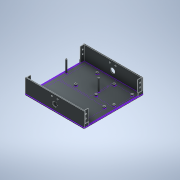
# Autodesk Inventor part: Lower_Housing
Saved by Autodesk Inventor 2022 (Build 260153000, 153)
## iProperties
Created: 2022-03-06
Part Number: Lower_Housing
Material: Iron, Cast
Document SubType Name: Modeling
Designer: Hajar
Density: 7.15 g/cm^3
Appearance: Iron Gray
Author: Hajar
Autodesk Inventor part; units mm, degrees
ref_plane "YZ Plane" through (0, 0, 0) normal (1, 0, 0) x (0, 1, 0)
ref_plane "XZ Plane" through (0, 0, 0) normal (0, 1, 0) x (-1, 0, 0)
ref_plane "XY Plane" through (0, 0, 0) normal (0, 0, 1) x (1, 0, 0)
sketch "Sketch1" plane through (0, 0, 0) normal (0, 1, 0) x (-1, 0, 0)
  line L0 (101.0364, -60.995) -> (-18.9636, -60.995)
  line L1 (-18.9636, -60.995) -> (-18.9636, 59.005)
  line L2 (-18.9636, 59.005) -> (101.0364, 59.005)
  line L3 (101.0364, 59.005) -> (101.0364, -60.995)
  line L4 (93.1598, 54.938) -> (-8.3402, 54.938) construction
  line L5 (-8.3402, 54.938) -> (-8.3402, 1.138) construction
  line L6 (-8.3402, 1.138) -> (93.1598, 1.138) construction
  line L7 (93.1598, 1.138) -> (93.1598, 54.938) construction
  line L8 (92.9387, -1.5201) -> (30.3387, -1.5201) construction
  line L9 (30.3387, -1.5201) -> (30.3387, -58.6201) construction
  line L10 (30.3387, -58.6201) -> (92.9387, -58.6201) construction
  line L11 (92.9387, -58.6201) -> (92.9387, -1.5201) construction
  line L12 (27.7395, -7.49) -> (-15.5605, -7.49) construction
  line L13 (-15.5605, -7.49) -> (-15.5605, -50.79) construction
  line L14 (-15.5605, -50.79) -> (27.7395, -50.79) construction
  line L15 (27.7395, -50.79) -> (27.7395, -7.49) construction
  line L16 (65.0387, -49.7201) -> (62.2387, -49.7201) construction
  line L17 (62.2387, -49.7201) -> (62.2387, -52.5201) construction
  line L18 (62.2387, -52.5201) -> (65.0387, -52.5201) construction
  line L19 (65.0387, -52.5201) -> (65.0387, -49.7201) construction
  circle A0 centre (65.0387, -7.1201) radius 1.4
  circle A1 centre (63.6387, -51.1201) radius 1.4
  line L20 (92.1598, 53.938) -> (89.3598, 53.938) construction
  line L21 (89.3598, 53.938) -> (89.3598, 51.138) construction
  line L22 (89.3598, 51.138) -> (92.1598, 51.138) construction
  line L23 (92.1598, 51.138) -> (92.1598, 53.938) construction
  line L24 (-4.5402, 4.938) -> (-7.3402, 4.938) construction
  line L25 (-7.3402, 4.938) -> (-7.3402, 2.138) construction
  line L26 (-7.3402, 2.138) -> (-4.5402, 2.138) construction
  line L27 (-4.5402, 2.138) -> (-4.5402, 4.938) construction
  circle A2 centre (-5.9402, 3.538) radius 1.4
  circle A3 centre (90.7598, 52.538) radius 1.4
  line L28 (26.3395, -8.59) -> (23.5395, -8.59) construction
  line L29 (23.5395, -8.59) -> (23.5395, -11.39) construction
  line L30 (23.5395, -11.39) -> (26.3395, -11.39) construction
  line L31 (26.3395, -11.39) -> (26.3395, -8.59) construction
  line L32 (-11.3605, -46.89) -> (-14.1605, -46.89) construction
  line L33 (-14.1605, -46.89) -> (-14.1605, -49.69) construction
  line L34 (-14.1605, -49.69) -> (-11.3605, -49.69) construction
  line L35 (-11.3605, -49.69) -> (-11.3605, -46.89) construction
  line L36 (-11.3605, -8.59) -> (-14.1605, -8.59) construction
  line L37 (-14.1605, -8.59) -> (-14.1605, -11.39) construction
  line L38 (-14.1605, -11.39) -> (-11.3605, -11.39) construction
  line L39 (-11.3605, -11.39) -> (-11.3605, -8.59) construction
  line L40 (26.3395, -46.89) -> (23.5395, -46.89) construction
  line L41 (23.5395, -46.89) -> (23.5395, -49.69) construction
  line L42 (23.5395, -49.69) -> (26.3395, -49.69) construction
  line L43 (26.3395, -49.69) -> (26.3395, -46.89) construction
  circle A4 centre (24.9395, -9.99) radius 1.4
  circle A5 centre (24.9395, -48.29) radius 1.4
  circle A6 centre (-12.7605, -48.29) radius 1.4
  circle A7 centre (-12.7605, -9.99) radius 1.4
  circle A8 centre (24.9395, -9.99) radius 2.4
  circle A9 centre (24.9395, -48.29) radius 2.4
  circle A10 centre (-12.7605, -48.29) radius 2.4
  circle A11 centre (-12.7605, -9.99) radius 2.4
  circle A12 centre (63.6387, -51.1201) radius 2.4
  circle A13 centre (65.0387, -7.1201) radius 2.4
  circle A14 centre (-5.9402, 3.538) radius 2.4
  circle A15 centre (90.7598, 52.538) radius 2.4
  line L44 (-20.9636, 61.005) -> (103.0364, 61.005)
  line L45 (103.0364, 61.005) -> (103.0364, -62.995)
  line L46 (103.0364, -62.995) -> (-20.9636, -62.995)
  line L47 (-20.9636, -62.995) -> (-20.9636, 61.005)
  circle A16 centre (97.4742, -19.995) radius 1.4
  circle A17 centre (97.4742, 57.3306) radius 1.4
  circle A18 centre (53.0364, 57.3306) radius 1.4
  circle A19 centre (29.2299, -19.995) radius 1.4
  circle A20 centre (29.0364, 57.3306) radius 1.4
  dimension "d0" = 120
  dimension "d1" = 120
  dimension "d8" = 101.5
  dimension "d9" = 53.8
  dimension "d10" = 62.6
  dimension "d11" = 57.1
  dimension "d12" = 43.3
  dimension "d13" = 43.3
  dimension "d24" = 4.067
  dimension "d25" = 10.6234
  dimension "d27" = 10.205
  dimension "d28" = 3.403
  dimension "d29" = 2.3749
  dimension "d30" = 8.0977
  dimension "d39" = 2.8
  dimension "d40" = 2.8
  dimension "d41" = 6.1
  dimension "d42" = 2.8
  dimension "d43" = 2.8
  dimension "d44" = 2.8
  dimension "d45" = 2.8
  dimension "d46" = 1
  dimension "d47" = 1
  dimension "d48" = 1
  dimension "d49" = 1
  dimension "d50" = 2.8
  dimension "d51" = 2.8
  dimension "d52" = 2.8
  dimension "d53" = 2.8
  dimension "d54" = 2.8
  dimension "d55" = 2.8
  dimension "d56" = 2.8
  dimension "d57" = 2.8
  dimension "d58" = 1.4
  dimension "d59" = 1.1
  dimension "d60" = 1.4
  dimension "d61" = 1.1
  dimension "d62" = 1.1
  dimension "d63" = 1.4
  dimension "d64" = 1.1
  dimension "d65" = 1.4
  dimension "d66" = 4.8
  dimension "d67" = 4.8
  dimension "d68" = 4.8
  dimension "d69" = 4.8
  dimension "d70" = 4.8
  dimension "d71" = 4.8
  dimension "d72" = 4.8
  dimension "d73" = 4.8
  dimension "d74" = 124
  dimension "d75" = 124
  dimension "d76" = 2
  dimension "d77" = 2
  dimension "d144" = 44
  dimension "d145" = 2.8
  dimension "d146" = 41
  dimension "d148" = 2.8
  dimension "d149" = 2.8
  dimension "d150" = 50
  dimension "d154" = 2.8
  dimension "d155" = 50
  constraints: 96 end point, 24 parallel, 21 centre point, 10 horizontal, 10 perpendicular, 8 coincident, 3 tangent, 2 point on line
  measures "d0" distance of L1.end L2.end
  measures "d1" distance of L0.end L1.end
  measures "d8" distance of L6.end L5.end
  measures "d9" distance of L5.end L4.end
  measures "d10" distance of L10.end L9.end
  measures "d11" distance of L9.end L8.end
  measures "d12" distance of L14.end L13.end
  measures "d13" distance of L13.end L12.end
  measures "d24" distance between parallel lines of L2 L4
  measures "d25" distance between parallel lines of L1 L5
  measures "d27" distance between parallel lines of L0 L14
  measures "d28" distance between parallel lines of L1 L13
  measures "d29" distance between parallel lines of L0 L10
  measures "d30" distance between parallel lines of L3 L11
  measures "d39" distance of L18.end L17.end
  measures "d40" distance of L17.end L16.end
  measures "d41" distance between parallel lines of L10 L18
  measures "d42" distance of L22.end L21.end
  measures "d43" distance of L21.end L20.end
  measures "d44" distance of L26.end L25.end
  measures "d45" distance of L25.end L24.end
  measures "d46" distance between parallel lines of L4 L20
  measures "d47" distance between parallel lines of L7 L23
  measures "d48" distance between parallel lines of L6 L26
  measures "d49" distance between parallel lines of L5 L25
  measures "d50" distance of L30.end L29.end
  measures "d51" distance of L29.end L28.end
  measures "d52" distance of L34.end L33.end
  measures "d53" distance of L33.end L32.end
  measures "d54" distance of L38.end L37.end
  measures "d55" distance of L37.end L36.end
  measures "d56" distance of L42.end L41.end
  measures "d57" distance of L41.end L40.end
  measures "d58" distance between parallel lines of L13 L37
  measures "d59" distance between parallel lines of L12 L36
  measures "d60" distance between parallel lines of L13 L33
  measures "d61" distance between parallel lines of L14 L34
  measures "d62" distance between parallel lines of L12 L28
  measures "d63" distance between parallel lines of L15 L31
  measures "d64" distance between parallel lines of L14 L42
  measures "d65" distance between parallel lines of L15 L43
  measures "d66" diameter of A8
  measures "d67" diameter of A9
  measures "d68" diameter of A10
  measures "d69" diameter of A11
  measures "d70" diameter of A12
  measures "d71" diameter of A13
  measures "d72" diameter of A14
  measures "d73" diameter of A15
  measures "d74" distance of L45.end L46.end
  measures "d75" distance of L44.end L45.end
  measures "d76" distance between parallel lines of L44 L2
  measures "d77" distance between parallel lines of L47 L1
  measures "d144" vertical distance of A0.centre A1.centre
  measures "d145" diameter of A16
  measures "d146" distance from line of A16.centre L0
  measures "d148" diameter of A17
  measures "d149" diameter of A18
  measures "d150" distance from line of L45 A18.centre
  measures "d154" diameter of A20
  measures "d155" distance from line of L47 A20.centre
extrude "Extrusion1" add sketch "Sketch1" against normal blind 2.5 contours L0 L1 L2 L3 | A0 | A1 | A2 | A3 | A4 | A5 | A6 | A7 | A8 | A9 | A10 | A11 | A12 | A13 | A14 | A15 | L44 L45 L46 L47 | A16 | A17 | A18 | A19 | A20
extrude "Extrusion2" add sketch "Sketch1" along normal blind 30 contours L44 L45 L46 L47
extrude "Extrusion3" add sketch "Sketch1" along normal blind 3 contours A15
extrude "Extrusion4" add sketch "Sketch1" along normal blind 3 contours A13
extrude "Extrusion5" add sketch "Sketch1" along normal blind 3 contours A12
extrude "Extrusion6" add sketch "Sketch1" along normal blind 3 contours A9
extrude "Extrusion7" add sketch "Sketch1" along normal blind 3 contours A8
extrude "Extrusion8" add sketch "Sketch1" along normal blind 3 contours A14
extrude "Extrusion9" add sketch "Sketch1" along normal blind 3 contours A11
extrude "Extrusion10" add sketch "Sketch1" along normal blind 3 contours A10
sketch "Sketch3" plane through (-103.0364, -2.5, -62.995) normal (-1, 0, 0) x (0, 0, 1)
  line L0 (122, 32.5) -> (2, 32.5) projected
  line L1 (2, 2.5) -> (122, 2.5) projected
  line L2 (10, 32.5) -> (114, 32.5)
  line L3 (114, 32.5) -> (114, 2.5)
  line L4 (114, 2.5) -> (10, 2.5)
  line L5 (10, 2.5) -> (10, 32.5)
  line L6 (0, 0) -> (0, 32.5) projected
  point P0 (62.995, 2.5)
  dimension "d98" = 104
  dimension "d99" = 10
  constraints: 8 end point, 2 parallel, 2 point on line, 1 horizontal, 1 perpendicular
  measures "d98" distance of L3.end L4.end
  measures "d99" distance from line of L6 L2.start
extrude "Extrusion11" cut sketch "Sketch3" against normal blind 3
sketch "Sketch4" plane through (20.9636, -2.5, 61.005) normal (1, 0, 0) x (0, 0, -1)
  line L0 (122, 32.5) -> (2, 32.5) projected
  line L1 (10, 32.5) -> (114, 32.5)
  line L2 (114, 32.5) -> (114, 2.5)
  line L3 (114, 2.5) -> (10, 2.5)
  line L4 (10, 2.5) -> (10, 32.5)
  line L5 (0, 0) -> (0, 32.5) projected
  point P0 (61.005, 2.5)
  dimension "d102" = 104
  dimension "d103" = 10
  constraints: 8 end point, 2 parallel, 1 horizontal, 1 perpendicular, 1 point on line
  measures "d102" distance of L2.end L3.end
  measures "d103" distance between parallel lines of L5 L4
extrude "Extrusion12" cut sketch "Sketch4" against normal blind 3
sketch "Sketch5" plane through (20.9636, -2.5, 61.005) normal (1, 0, 0) x (0, 0, -1)
  line L0 (3.7, 25.8817) -> (6.5, 25.8817) construction
  line L1 (6.5, 25.8817) -> (6.5, 23.0817) construction
  line L2 (6.5, 23.0817) -> (3.7, 23.0817) construction
  line L3 (3.7, 23.0817) -> (3.7, 25.8817) construction
  line L4 (3.7, 17.6669) -> (6.5, 17.6669) construction
  line L5 (6.5, 17.6669) -> (6.5, 14.8669) construction
  line L6 (6.5, 14.8669) -> (3.7, 14.8669) construction
  line L7 (3.7, 14.8669) -> (3.7, 17.6669) construction
  line L8 (10, 2.5) -> (10, 32.5) projected
  circle A0 centre (5.1, 24.8) radius 1.4
  circle A1 centre (5.1, 16.3) radius 1.4
  line L9 (117.5, 24.7669) -> (120.3, 24.7669) construction
  line L10 (0, 32.5) -> (10, 32.5) projected
  line L11 (117.5, 16.3) -> (120.3, 16.3) construction
  line L12 (114, 32.5) -> (114, 2.5) projected
  circle A2 centre (118.9, 24.8) radius 1.4
  circle A3 centre (118.9, 16.3) radius 1.4
  line L13 (114, 32.5) -> (124, 32.5) projected
  point P0 (61.005, 2.5)
  dimension "d106" = 2.8
  dimension "d107" = 2.8
  dimension "d108" = 2.8
  dimension "d109" = 2.8
  dimension "d110" = 3.5
  dimension "d111" = 3.5
  dimension "d112" = 8.5
  dimension "d115" = 7.7
  dimension "d120" = 7.7
  dimension "d121" = 8.5
  dimension "d122" = 2.8
  dimension "d123" = 2.8
  dimension "d124" = 4.9
  dimension "d125" = 4.9
  dimension "d126" = 4.9
  dimension "d127" = 4.9
  constraints: 20 end point, 4 centre point, 4 parallel, 3 horizontal, 1 perpendicular
  measures "d106" distance of L1.end L2.end
  measures "d107" distance of L0.end L1.end
  measures "d108" distance of L5.end L6.end
  measures "d109" distance of L4.end L5.end
  measures "d110" distance between parallel lines of L8 L5
  measures "d111" distance between parallel lines of L8 L1
  measures "d112" distance of A1.centre A0.centre
  measures "d115" distance from line of L10 A0.centre
  measures "d120" distance from line of L13 A2.centre
  measures "d121" distance of A3.centre A2.centre
  measures "d122" diameter of A2
  measures "d123" diameter of A3
  measures "d124" distance from line of L12 A2.centre
  measures "d125" distance from line of L12 A3.centre
  measures "d126" distance from line of L8 A1.centre
  measures "d127" distance from line of L8 A0.centre
extrude "Extrusion13" cut sketch "Sketch5" against normal blind 130
sketch "Sketch6" plane through (-103.0364, -2.5, 61.005) normal (0, 0, 1) x (1, 0, 0)
  line L0 (57, 19.5) -> (67, 19.5) construction
  line L1 (67, 19.5) -> (67, 9.5) construction
  line L2 (67, 9.5) -> (57, 9.5) construction
  line L3 (57, 9.5) -> (57, 19.5) construction
  line L4 (0, 32.5) -> (124, 32.5) projected
  line L5 (54.55, 28) -> (57.35, 28) construction
  line L6 (57.35, 28) -> (57.35, 25.2) construction
  line L7 (57.35, 25.2) -> (54.55, 25.2) construction
  line L8 (54.55, 25.2) -> (54.55, 28) construction
  line L9 (66.65, 25.1915) -> (69.45, 25.1915) construction
  line L10 (69.45, 25.1915) -> (69.45, 27.9915) construction
  line L11 (69.45, 27.9915) -> (66.65, 27.9915) construction
  line L12 (66.65, 27.9915) -> (66.65, 25.1915) construction
  line L13 (124, 0) -> (124, 32.5) projected
  line L14 (0, 0) -> (0, 32.5) projected
  circle A0 centre (55.95, 26.5915) radius 1.4
  circle A1 centre (68.05, 26.5915) radius 1.4
  circle A2 centre (62, 14.5) radius 5
  point P0 (103.0364, 2.5)
  dimension "d130" = 10
  dimension "d131" = 10
  dimension "d132" = 13
  dimension "d133" = 2.8
  dimension "d134" = 2.8
  dimension "d135" = 2.8
  dimension "d136" = 2.8
  dimension "d137" = 9.3
  dimension "d138" = 5.7
  dimension "d139" = 54.55
  dimension "d140" = 54.55
  dimension "d141" = 57
  constraints: 24 end point, 6 parallel, 3 centre point, 2 horizontal, 2 perpendicular, 1 tangent
  measures "d130" distance of L1.end L2.end
  measures "d131" distance of L0.end L1.end
  measures "d132" distance between parallel lines of L4 L0
  measures "d133" distance of L6.end L7.end
  measures "d134" distance of L5.end L6.end
  measures "d135" distance of L11.end L10.end
  measures "d136" distance of L10.end L9.end
  measures "d137" distance between parallel lines of L12 L6
  measures "d138" distance between parallel lines of L0 L7
  measures "d139" distance between parallel lines of L13 L10
  measures "d140" distance between parallel lines of L14 L8
  measures "d141" distance between parallel lines of L13 L1
extrude "Extrusion14" cut sketch "Sketch6" against normal blind 130
extrude "Extrusion15" add sketch "Sketch1" along normal blind 26 contours A16 | A17 | A18 | A19
sketch "Sketch7" plane through (20.9636, -2.5, 61.005) normal (1, 0, 0) x (0, 0, -1)
  line L0 (2, 2.5) -> (2, 32.5) projected
  line L1 (10, 32.5) -> (10, 2.5) projected
  line L2 (2, 32.5) -> (10, 32.5)
  line L3 (10, 32.5) -> (10, 8.5)
  line L4 (10, 8.5) -> (2, 8.5)
  line L5 (2, 8.5) -> (2, 32.5)
  line L6 (122, 32.5) -> (114, 32.5) projected
  line L7 (122, 2.5) -> (122, 32.5) projected
  line L8 (114, 32.5) -> (122, 32.5)
  line L9 (122, 32.5) -> (122, 8.5)
  line L10 (122, 8.5) -> (114, 8.5)
  line L11 (114, 8.5) -> (114, 32.5)
  point P0 (61.005, 2.5)
  dimension "d156" = 24
  dimension "d157" = 24
  constraints: 16 end point, 4 parallel, 2 horizontal, 2 perpendicular, 2 point on line
  measures "d156" distance of L2.end L3.end
  measures "d157" distance of L8.end L9.end
extrude "Extrusion16" cut sketch "Sketch7" against normal blind 1
sketch "Sketch8" plane through (-103.0364, -2.5, -62.995) normal (-1, 0, 0) x (0, 0, 1)
  line L0 (2, 2.5) -> (2, 32.5) projected
  line L1 (10, 2.5) -> (10, 32.5) projected
  line L2 (2, 32.5) -> (10, 32.5)
  line L3 (10, 32.5) -> (10, 8.5)
  line L4 (10, 8.5) -> (2, 8.5)
  line L5 (2, 8.5) -> (2, 32.5)
  line L6 (114, 32.5) -> (124, 32.5) projected
  line L7 (122, 2.5) -> (122, 32.5) projected
  line L8 (114, 32.5) -> (122, 32.5)
  line L9 (122, 32.5) -> (122, 8.5)
  line L10 (122, 8.5) -> (114, 8.5)
  line L11 (114, 8.5) -> (114, 32.5)
  point P0 (62.995, 2.5)
  dimension "d160" = 24
  dimension "d161" = 24
  constraints: 16 end point, 4 parallel, 2 horizontal, 2 perpendicular, 2 point on line
  measures "d160" distance of L2.end L3.end
  measures "d161" distance of L8.end L9.end
extrude "Extrusion17" cut sketch "Sketch8" against normal blind 1
extrude "Extrusion18" cut sketch "Sketch1" against normal blind 1.5 contours A0 | A1 | A2 | A3 | A4 | A5 | A6 | A7
body "Solid1"
